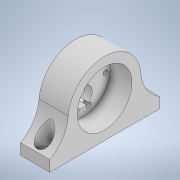
# Autodesk Inventor part: Motor Mount V2
Saved by Autodesk Inventor 2020 (Build 240168000, 168)
## iProperties
Created: 2020-01-13
Part Number: Motor Mount V2
Material: Generic
Document SubType Name: Modeling
Designer: maple
Density: 1 g/cm^3
Appearance: Default
Author: maple
Autodesk Inventor part; units mm, degrees
ref_plane "YZ Plane" through (0, 0, 0) normal (1, 0, 0) x (0, 1, 0)
ref_plane "XZ Plane" through (0, 0, 0) normal (0, 1, 0) x (-1, 0, 0)
ref_plane "XY Plane" through (0, 0, 0) normal (0, 0, 1) x (1, 0, 0)
sketch "Sketch1" plane through (0, 0, 0) normal (0, 1, 0) x (-1, 0, 0)
  line L0 (0, 0) -> (-20.32, 0)
  line L1 (-20.32, 0) -> (-20.32, -76.2)
  line L2 (-20.32, -76.2) -> (0, -76.2)
  line L3 (0, -76.2) -> (0, 0)
  dimension "d0" = 20.32
  dimension "d1" = 76.2
  constraints: 8 end point, 2 parallel, 1 horizontal, 1 perpendicular
  measures "d0" distance of L2.end L1.end
  measures "d1" distance of L1.end L0.end
extrude "Extrusion1" add sketch "Sketch1" along normal blind 7.62
sketch "Sketch2" plane through (0, 7.62, 0) normal (0, 1, 0) x (1, 0, 0)
  line L0 (0, 0) -> (0, 12.7)
  line L1 (0, 12.7) -> (20.32, 12.7)
  line L2 (20.32, 12.7) -> (20.32, 63.5)
  line L3 (20.32, 63.5) -> (0, 63.5)
  line L4 (0, 63.5) -> (0, 12.7)
  dimension "d4" = 12.7
  dimension "d5" = 20.32
  dimension "d6" = 50.8
  constraints: 10 end point, 2 parallel, 1 horizontal, 1 perpendicular, 1 vertical
  measures "d4" distance of L0.start L0.end
  measures "d5" distance of L3.end L2.end
  measures "d6" distance of L2.end L1.end
extrude "Extrusion2" add sketch "Sketch2" along normal blind 43.18
sketch "Sketch3" plane through (20.32, 0, 0) normal (1, 0, 0) x (0, 0, -1)
  line L0 (12.7, 50.8) -> (63.5, 50.8) projected
  line L1 (38.1, 50.8) -> (38.1, 25.4)
  circle A0 centre (38.1, 25.4) radius 19.05
  point P0 (0, 0)
  dimension "d9" = 25.4
  dimension "d10" = 38.1
  constraints: 2 end point, 1 centre point, 1 coincident, 1 midpoint, 1 vertical
  measures "d9" distance of L1.start L1.end
  measures "d10" diameter of A0
extrude "Extrusion3" cut sketch "Sketch3" against normal blind 15.24
fillet "Fillet1" radius 25.4 2 edges at (10.16, 50.8, -63.5) (10.16, 50.8, -12.7)
sketch "Sketch6" plane through (0, 7.62, 0) normal (0, 1, 0) x (1, 0, 0)
  line L0 (0, 0) -> (20.32, 0) projected
  line L1 (10.16, 0) -> (10.16, 6.35)
  line L2 (20.32, 76.2) -> (0, 76.2) projected
  line L3 (10.16, 76.2) -> (10.16, 69.85)
  dimension "d20" = 6.35
  dimension "d21" = 6.35
  constraints: 4 end point, 2 midpoint, 2 vertical
  measures "d20" distance of L1.start L1.end
  measures "d21" distance of L3.start L3.end
fillet "Fillet2" radius 25.4 2 edges at (10.16, 7.62, -63.5) (10.16, 7.62, -12.7)
hole "Hole1" at (10.16, 7.62, -6.35) at (10.16, 7.62, -69.85) direction (0, -1, 0) diameter 5.08 end through all counterbore diameter 10.16 counterbore depth 3.81
sketch "Sketch7" plane through (10.16, 7.62, -6.35) normal (0, -1, 0) x (1, 0, 0)
  circle A0 centre (0, 0) radius 5.08
  circle A1 centre (0, -63.5) radius 2.54 projected
  line L0 (-2.54, -63.5) -> (0, -63.5)
  circle A2 centre (0, -63.5) radius 5.08
  point P0 (-10.16, 6.35)
  dimension "d30" = 10.16
  dimension "d31" = 10.16
  constraints: 2 centre point, 2 end point, 1 coincident, 1 horizontal, 1 horizontal alignment, 1 other
  measures "d30" diameter of A0
  measures "d31" diameter of A2
extrude "Extrusion5" cut sketch "Sketch7" against normal blind 15.24 contours A0 | A1 | A2
sketch "Sketch9" plane through (5.08, 25.4, -38.1) normal (1, 0, 0) x (0, 0, -1)
  line L0 (0, 0) -> (0, -6.604)
  circle A0 centre (0, -6.604) radius 6.604
  line L1 (0, -6.604) -> (-3.302, -12.3232)
  line L2 (0, -6.604) -> (6.604, -6.604) construction
  line L3 (0, -6.604) -> (3.302, -12.3232)
  line L4 (0, -6.604) -> (6.604, -6.604) construction
  line L5 (-3.302, -12.3232) -> (-4.064, -13.6431)
  line L6 (3.302, -12.3232) -> (4.064, -13.6431)
  line L7 (3.302, -12.3232) -> (4.826, -12.3232) construction
  circle A1 centre (-4.064, -13.6431) radius 1.778
  circle A2 centre (4.064, -13.6431) radius 1.778
  circle A3 centre (0, 0) radius 19.05 projected
  line L8 (-19.05, 0) -> (-17.526, 0)
  line L9 (-17.526, 0) -> (-15.875, 0)
  circle A4 centre (-15.875, 0) radius 1.651
  line L10 (19.05, 0) -> (17.526, 0)
  line L11 (17.526, 0) -> (15.875, 0)
  circle A5 centre (15.875, 0) radius 1.651
  line L12 (0, 0) -> (-9.525, 16.4978)
  line L13 (0, 0) -> (9.525, 16.4978)
  line L14 (-9.525, 16.4978) -> (-8.763, 15.178)
  line L15 (-8.763, 15.178) -> (-7.9375, 13.7482)
  line L16 (9.525, 16.4978) -> (8.763, 15.178)
  line L17 (8.763, 15.178) -> (7.9375, 13.7482)
  circle A6 centre (-7.9375, 13.7482) radius 1.651
  circle A7 centre (7.9375, 13.7482) radius 1.651
  point P0 (-38.1, -25.4)
  point P1 (-2.5627, -12.6905)
  point P2 (2.5627, -12.6905)
  point P3 (3.9897, -11.8666)
  point P4 (-3.9897, -11.8666)
  dimension "d47" = 6.604
  dimension "d48" = 120
  dimension "d49" = 60
  dimension "d50" = 1.524
  dimension "d51" = 1.524
  dimension "d52" = 60
  dimension "d53" = 3.556
  dimension "d54" = 3.556
  dimension "d55" = 1.524
  dimension "d56" = 1.651
  dimension "d57" = 1.524
  dimension "d58" = 1.651
  dimension "d59" = 1.524
  dimension "d60" = 1.651
  dimension "d61" = 1.524
  dimension "d62" = 1.651
  constraints: 36 end point, 8 point on circle, 7 coincident, 6 horizontal, 5 point on line, 3 centre point, 3 equal length, 2 horizontal alignment, 1 vertical, 10 other
  measures "d47" distance of L0.start L0.end
  measures "d48" angle of L1 L2
  measures "d49" angle of L3 L4
  measures "d50" distance of L1.end L5.end
  measures "d51" distance of L3.end L6.end
  measures "d52" angle of L6 L7
  measures "d53" diameter of A1
  measures "d54" diameter of A2
  measures "d55" distance of L8.start L8.end
  measures "d56" distance of L8.end L9.end
  measures "d57" distance of L10.start L10.end
  measures "d58" distance of L10.end L11.end
  measures "d59" distance of L12.end L14.end
  measures "d60" distance of L14.end L15.end
  measures "d61" distance of L13.end L16.end
  measures "d62" distance of L16.end L17.end
extrude "Extrusion7" cut sketch "Sketch9" against normal blind 25.4 contours A0 A2 L3 L0 | L0 L1 A1 A0 | L3 A2 A0 A1 L1 | A1 L1 A0 | A0 A1 | A6 L12 | L12 A6 | A7 L13 | L13 A7 | A1 A0 L1 | A2 A0 L3 | L3 A0 A2 | A2 A0 | A4 | A5
body "Solid1"
